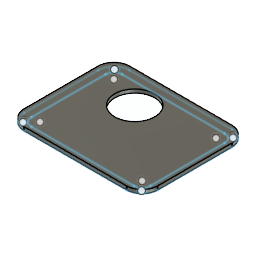
Top_Cover (Autodesk Fusion 360 design; units mm, degrees)
part number: 2026-06-20-23-45-20-806
Autodesk Fusion 360 part; units mm, degrees
sketch "Top cover" plane through (0, 0, 0) normal (0, 0, 1) x (1, 0, 0)
  line L0 (-42.5673, 50.8332) -> (-42.5673, -20.4349)
  line L1 (86.2077, 50.8332) -> (86.2042, 51.2331)
  line L2 (-42.5637, 51.2331) -> (-42.5673, 50.8332)
  line L3 (-27.4488, 65.9517) -> (-27.8488, 65.9481)
  arc A0 (-42.5637, -20.8348) -> (-27.8488, -35.5498) centre (-27.4173, -20.4033) ccw
  line L4 (-27.4488, -35.5533) -> (71.0893, -35.5533)
  arc A1 (-27.8488, 65.9481) -> (-42.5637, 51.2331) centre (-27.4173, 50.8017) ccw
  line L5 (-27.8488, -35.5498) -> (-27.4488, -35.5533)
  line L6 (71.0893, -35.5533) -> (71.4892, -35.5498)
  arc A2 (86.2042, 51.2331) -> (71.4892, 65.9481) centre (71.0577, 50.8017) ccw
  line L7 (71.4892, 65.9481) -> (71.0893, 65.9517)
  arc A3 (71.4892, -35.5498) -> (86.2042, -20.8348) centre (71.0577, -20.4033) ccw
  line L8 (71.0893, 65.9517) -> (-27.4488, 65.9517)
  line L9 (-42.5673, -20.4349) -> (-42.5637, -20.8348)
  line L10 (86.2042, -20.8348) -> (86.2077, -20.4349)
  line L11 (86.2077, -20.4349) -> (86.2077, 50.8332)
  arc A4 (79.1351, -20.6918) -> (71.3462, -28.4808) centre (71.0577, -20.4033) cw
  line L12 (71.3462, -28.4808) -> (71.0577, -28.4833)
  arc A5 (-27.7058, -28.4808) -> (-35.4947, -20.6918) centre (-27.4173, -20.4033) cw
  line L13 (-35.4973, -20.4033) -> (-35.4973, 50.8017)
  arc A6 (-35.4947, 51.0902) -> (-27.7058, 58.8791) centre (-27.4173, 50.8017) cw
  arc A7 (71.3462, 58.8791) -> (79.1351, 51.0902) centre (71.0577, 50.8017) cw
  line L14 (79.1351, 51.0902) -> (79.1377, 50.8017)
  line L15 (71.0577, 58.8817) -> (71.3462, 58.8791)
  line L16 (71.0577, -28.4833) -> (-27.4173, -28.4833)
  line L17 (-27.7058, 58.8791) -> (-27.4173, 58.8817)
  line L18 (-35.4973, 50.8017) -> (-35.4947, 51.0902)
  line L19 (-27.4173, 58.8817) -> (71.0577, 58.8817)
  line L20 (79.1377, 50.8017) -> (79.1377, -20.4033)
  line L21 (-35.4947, -20.6918) -> (-35.4973, -20.4033)
  line L22 (79.1377, -20.4033) -> (79.1351, -20.6918)
  line L23 (-27.4173, -28.4833) -> (-27.7058, -28.4808)
  circle A8 centre (78.9656, -28.8671) radius 2.45
  circle A9 centre (78.9656, 59.2655) radius 2.45
  circle A10 centre (-35.3252, -28.8671) radius 2.45
  circle A11 centre (-35.3252, 59.2655) radius 2.45
  line L24 (-35.4973, -20.4033) -> (-35.4947, -20.6918)
  line L25 (-35.4973, 50.8017) -> (-35.4973, -20.4033)
  line L26 (-27.7058, -28.4808) -> (-27.4173, -28.4833)
  line L27 (79.1351, -20.6918) -> (79.1377, -20.4033)
  line L28 (71.3462, 58.8791) -> (71.0577, 58.8817)
  arc A12 (79.1351, 51.0902) -> (71.3462, 58.8791) centre (71.0577, 50.8017) ccw
  line L29 (-35.4947, 51.0902) -> (-35.4973, 50.8017)
  line L30 (71.0577, 58.8817) -> (-27.4173, 58.8817)
  line L31 (-27.4173, 58.8817) -> (-27.7058, 58.8791)
  line L32 (79.1377, -20.4033) -> (79.1377, 50.8017)
  line L33 (79.1377, 50.8017) -> (79.1351, 51.0902)
  line L34 (71.0577, -28.4833) -> (71.3462, -28.4808)
  line L35 (-27.4173, -28.4833) -> (71.0577, -28.4833)
  arc A13 (-35.4947, -20.6918) -> (-27.7058, -28.4808) centre (-27.4173, -20.4033) ccw
  arc A14 (-27.7058, 58.8791) -> (-35.4947, 51.0902) centre (-27.4173, 50.8017) ccw
  arc A15 (71.3462, -28.4808) -> (79.1351, -20.6918) centre (71.0577, -20.4033) ccw
  circle A16 centre (-35.3252, 59.2655) radius 2.45
  circle A17 centre (-35.3252, 59.2655) radius 1.65
  circle A18 centre (-35.3252, -28.8671) radius 1.65
  circle A19 centre (-35.3252, -28.8671) radius 2.45
  circle A20 centre (78.9656, -28.8671) radius 1.65
  circle A21 centre (78.9656, 59.2655) radius 2.45
  circle A22 centre (78.9656, 59.2655) radius 1.65
  circle A23 centre (-35.3252, -28.8671) radius 2.8
  circle A24 centre (78.9656, -28.8671) radius 2.8
  circle A25 centre (78.9656, 59.2655) radius 2.8
  circle A26 centre (-35.3252, 59.2655) radius 2.8
  point P0 (78.9656, -28.8671)
  dimension "d5" = 5.6
  dimension "d6" = 5.6
  dimension "d7" = 5.6
  dimension "d8" = 5.6
  constraint concentric A19 A23
  constraint concentric A8 A24
  constraint concentric A21 A25
  constraint concentric A16 A26
  measures "d5" diameter of A23
  measures "d6" diameter of A24
  measures "d7" diameter of A25
  measures "d8" diameter of A26
extrude "Extrude1" add sketch "Top cover" along normal blind 3 contours L0 L1 L2 L3 A0 L4 A1 L5 L6 A2 L7 A3 L8 L9 L10 L11 | A4 L12 A5 L13 A6 A7 L14 L15 L16 L17 L18 L19 L20 L21 L22 L23 L24 L25 L26 L27 L28 A12 L29 L30 L31 L32 L33 L34 L35 A13 A14 A15 | A8 | A9 A21 | A10 A19 | A11 A16 | A17 | A18 | A20 | A22 | A23 | A24 | A25 | A26
extrude "Extrude2" add 1 faces at (38.2432, 32.1167, 3) along direction (0, 0, 1) blind 0.5
extrude "Extrude3" cut sketch "Top cover" along normal blind 2.7 contours A8 | A9 A21 | A10 A19 | A11 A16 | A17 | A18 | A20 | A22 | A23 | A24 | A25 | A26
sketch "speaker" plane through (0, 0, 3.5) normal (0, 0, 1) x (1, 0, 0)
  circle A0 centre (7.845, 35.6627) radius 18.5447
  circle A1 centre (7.845, 35.6627) radius 19.2723
  circle A2 centre (7.845, 35.6627) radius 19.2723
  circle A3 centre (7.845, 35.6627) radius 20
extrude "Extrude4" cut sketch "speaker" against normal blind 5 contours A0 | A1 A2
